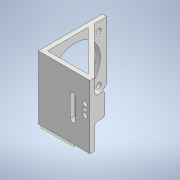
# Autodesk Inventor part: Bending Base
Saved by Autodesk Inventor 2022.2 (Build 262287000, 287)
## iProperties
Created: 2022-08-12
Part Number: Bending Base
Material: Generic
Document SubType Name: Modeling
Designer: Ilewicz
Density: 1 g/cm^3
Appearance: Default
Author: Ilewicz
Autodesk Inventor part; units mm, degrees
sketch "Sketch2" plane through (0, 0, 0) normal (1, 0, 0) x (0, 1, 0)
  line L0 (21.15, -4.6284) -> (21.15, -37.6716) projected
  line L1 (17.5822, -41.3607) -> (20.2107, -38.7322) projected
  arc A0 (20.2107, -38.7322) -> (20.65, -37.6716) centre (19.15, -37.6716) ccw projected
  line L2 (20.65, -37.6716) -> (20.65, -4.6284) projected
  arc A1 (20.65, -4.6284) -> (20.2107, -3.5678) centre (19.15, -4.6284) ccw projected
  line L3 (20.2107, -3.5678) -> (17.5822, -0.9393) projected
  arc A2 (17.5822, -0.9393) -> (16.5216, -0.5) centre (16.5216, -2) ccw projected
  line L4 (16.5216, -0.5) -> (-16.5216, -0.5) projected
  arc A3 (-16.5216, -0.5) -> (-17.5822, -0.9393) centre (-16.5216, -2) ccw projected
  line L5 (-17.5822, -0.9393) -> (-20.2107, -3.5678) projected
  arc A4 (-20.2107, -3.5678) -> (-20.65, -4.6284) centre (-19.15, -4.6284) ccw projected
  line L6 (-20.65, -4.6284) -> (-20.65, -37.6716) projected
  arc A5 (-20.65, -37.6716) -> (-20.2107, -38.7322) centre (-19.15, -37.6716) ccw projected
  line L7 (-20.2107, -38.7322) -> (-17.5822, -41.3607) projected
  arc A6 (-17.5822, -41.3607) -> (-16.5216, -41.8) centre (-16.5216, -40.3) ccw projected
  line L8 (-16.5216, -41.8) -> (16.5216, -41.8) projected
  arc A7 (16.5216, -41.8) -> (17.5822, -41.3607) centre (16.5216, -40.3) ccw projected
  circle A8 centre (0, -21.15) radius 16.5 projected
  circle A9 centre (15.5, -36.65) radius 1.55 projected
  circle A10 centre (-15.5, -36.65) radius 1.55 projected
  circle A11 centre (-15.5, -5.65) radius 1.55 projected
  circle A12 centre (15.5, -5.65) radius 1.55 projected
  line L9 (21.15, -37.6716) -> (21.15, -41.8)
  line L10 (21.15, -41.8) -> (15.1388, -41.8)
  line L11 (21.15, -4.6284) -> (21.15, -0.5)
  line L12 (-20.65, -4.7869) -> (-20.65, 0.2131)
  line L13 (-20.65, 0.2131) -> (21.15, 0.2131)
  line L14 (21.15, 0.2131) -> (21.15, -0.5)
  line L15 (-20.65, -4.7869) -> (-20.65, -4.6284)
  line L16 (21.15, -0.5) -> (20.65, -0.5)
  point P0 (0, 0)
  dimension "d2" = 5
  constraints: 16 end point, 3 vertical, 2 collinear, 2 point on line, 1 parallel
  measures "d2" distance of L12.start L12.end
extrude "Extrusion1" add sketch "Sketch2" along normal blind 3
sketch "Sketch5" plane through (3, 0, 0) normal (1, 0, 0) x (0, 0, -1)
  line L0 (41.8, 21.15) -> (-0.2131, 21.15) projected
  line L1 (-0.2131, -20.65) -> (37.6716, -20.65) projected
  line L2 (-0.2131, 21.15) -> (2.7869, 21.15)
  line L3 (2.7869, 21.15) -> (2.7869, -20.65)
  line L4 (2.7869, -20.65) -> (-0.2131, -20.65)
  line L5 (-0.2131, -20.65) -> (-0.2131, 21.15)
  point P0 (0, 0)
  dimension "d3" = 3
  constraints: 8 end point, 2 parallel, 1 horizontal, 1 perpendicular, 1 point on line
  measures "d3" distance of L3.end L4.end
ref_plane "Work Plane1" through (33.9341, -3.4404, -22.9827) normal (1, 0, 0) x (0, 1, 0)
extrude "Extrusion2" add sketch "Sketch5" along normal up to surface (30.9341 mm away)
sketch "Sketch12" plane through (0, 21.15, 0.2131) normal (0, 1, 0) x (1, 0, 0)
  line L0 (3, 3) -> (33.9341, 3) projected
  line L1 (29.6915, 3) -> (3, 29.6915)
  line L2 (3, 42.0131) -> (3, 3) projected
  line L3 (33.9341, 3) -> (3, 33.9341)
  line L4 (0, 42.0131) -> (0, 0) projected
  line L5 (0, 0) -> (33.9341, 0) projected
  line L6 (33.9341, 0) -> (33.9341, 3) projected
  line L7 (3, 3) -> (33.9341, 3) projected
  line L8 (3, 42.0131) -> (3, 3) projected
  line L9 (0, 42.0131) -> (3, 42.0131) projected
  point P0 (0, 0.2131)
  dimension "d25" = 3
  dimension "d26" = 45
  constraints: 4 end point, 3 point on line, 1 parallel
  measures "d25" distance between parallel lines of L1 L3
  measures "d26" angle of L2 L1
extrude "Extrusion7" add sketch "Sketch12" against normal blind 2 contours L0 L6 L5 L4 L9 L2 | L1 L2 L3 L0
ref_plane "Work Plane6" through (28.6495, -6.0754, -9.5607) normal (0, 0, 1) x (1, 0, 0)
sketch "Sketch7" plane through (3, -20.65, -2.7869) normal (0, 0, -1) x (-1, 0, 0)
  line L0 (-28.65, 23.05) -> (-28.65, 21.7895) projected
  arc A0 (-28.65, 23.05) -> (-28.25, 22.65) centre (-28.25, 23.05) ccw projected
  line L1 (-28.25, 22.65) -> (-25.65, 22.65) projected
  line L2 (-25.65, 15.5156) -> (-25.65, 22.65) projected
  line L3 (-25.65, 15.5156) -> (-27.64, 17.5537) projected
  line L4 (-27.64, 17.5537) -> (-27.65, 17.5537) projected
  line L5 (-29.9084, 20.2451) -> (-27.65, 17.5537) projected
  ellipse E0 centre (-29.15, 20.9127) end of major axis (-29.15, 19.8885) minor radius 1 (-30.15, 20.9127) -> (-29.9084, 20.2451) ccw projected
  line L6 (-30.15, 21.0006) -> (-30.15, 20.9127) projected
  line L7 (-30.15, 27.15) -> (-30.15, 21.0006) projected
  line L8 (-30.15, 27.15) -> (-28.65, 27.15) projected
  line L9 (-28.65, 21.7895) -> (-28.65, 27.15) projected
  line L10 (0, 0) -> (-30.9341, 0) projected
  line L11 (-25.65, 0) -> (-25.65, 41.8)
  line L12 (0, 41.8) -> (-30.9341, 41.8) projected
  line L13 (-30.9341, 39.8) -> (-30.9341, 0) projected
  line L14 (0, 0) -> (-30.9341, 0) projected
  line L15 (0, 41.8) -> (0, 0) projected
  line L16 (0, 41.8) -> (-26.6915, 41.8) projected
  circle A1 centre (-27.6209, 23.6216) radius 1.25
  circle A2 centre (-27.653, 20.3029) radius 1.5 projected
  circle A3 centre (-27.653, 26.8687) radius 1.5 projected
  line L17 (-26.6915, 41.8) -> (-26.6915, 39.8) projected
  line L18 (-26.6915, 39.8) -> (-30.9341, 39.8) projected
  line L19 (-30.9341, 2) -> (-30.9341, 0) projected
  line L20 (-30.9341, 41.8) -> (-30.9341, 39.8) projected
  line L21 (-25.65, 31.1874) -> (-30.9341, 31.1874)
  line L22 (-30.9341, 39.8) -> (-30.9341, 0) projected
  line L23 (-25.65, 16.0384) -> (-30.9341, 16.0384)
  point P0 (3, 20.65)
  point P1 (-30.9341, 19.4722)
  point P2 (-30.9341, 0)
  point P3 (-30.9341, 41.8)
  point P4 (-30.9341, 23.8955)
  point P5 (-30.9341, 19.4722)
  point P6 (-25.65, 15.5156)
  point P7 (-25.65, 22.65)
  point P8 (-25.65, 41.8)
  point P9 (-30.9341, 25.7096)
  point P10 (-30.9341, 17.4244)
  point P11 (-30.9341, 16.0384)
  point P12 (-25.65, 16.0384)
  point P13 (-26.1605, 16.0384)
  point P14 (-29.1264, 27.15)
  point P15 (-28.65, 25.748)
  point P16 (-28.65, 24.3312)
  point P17 (-26.8345, 22.65)
  dimension "d23" = 2.5
  constraints: 6 end point, 6 point on line, 2 perpendicular, 1 centre point, 1 collinear, 1 tangent, 1 vertical, 1 other
  measures "d23" diameter of A1
extrude "Extrusion3" add sketch "Sketch7" along normal up to surface (6.7738 mm away) contours A1 L1 L2 L23 L3 L4 L5 E0 L6 L7 L8 A3 L9 | L9 A3 L8 L7 L6 E0 L5 L4 L3 L23 L13 L21 L11 L1 A1
ref_plane "Work Plane5" through (3, -20.65, -9.2979) normal (0, 0, -1) x (-1, 0, 0)
sketch "Sketch10" plane through (0, -20.65, 0.2131) normal (0, 0, 1) x (1, 0, 0)
  circle A0 centre (22.5901, 16.9163) radius 1.59 projected
  circle A1 centre (22.5901, 25.2418) radius 1.59 projected
  line L0 (24.1801, 28.0246) -> (24.1801, 13.7754)
  line L1 (21.0001, 13.7754) -> (21.0001, 28.0246)
  arc A2 (21.0001, 13.7754) -> (24.1801, 13.7754) centre (22.5901, 13.7754) ccw
  line L2 (3, 0) -> (32.7496, 13.2856) projected
  arc A3 (24.1801, 28.0246) -> (21.0001, 28.0246) centre (22.5901, 28.0246) ccw
  line L3 (33.9341, 27.9855) -> (3, 41.8) projected
  point P0 (0, 20.65)
  point P1 (32.8942, 25.4407)
  point P2 (3, 41.8)
  point P3 (33.9341, 27.9855)
  dimension "d16" = 4.59
  dimension "d17" = 4.59
  constraints: 5 tangent, 4 end point, 4 point on circle, 2 centre point, 2 equal radius, 1 vertical, 1 other
  measures "d16" distance from line of L2 A2.centre
extrude "Extrusion5" cut sketch "Sketch10" against normal blind 10
ref_plane "Work Plane3" through (20.0901, -24.2569, 0.2131) normal (0, -1, 0) x (1, 0, 0)
sketch "Sketch14" plane through (33.9341, -20.65, 0.2131) normal (1, 0, 0) x (0, 0, -1)
  point P0 (0.2131, 20.65)
sketch "Sketch15" plane through (33.9341, -20.65, -9.5607) normal (0, 0, -1) x (-1, 0, 0)
  circle A0 centre (3.2811, 20.3029) radius 1.5 projected
  circle A1 centre (3.2811, 20.3029) radius 1.5 projected
  circle A2 centre (3.3132, 23.6216) radius 1.25 projected
  circle A3 centre (3.2811, 26.8687) radius 1.5 projected
  circle A4 centre (3.2811, 20.3029) radius 1.5 projected
  line L0 (0, 16.0384) -> (5.2841, 16.0384) projected
  line L1 (5.2841, 16.0384) -> (5.2841, 31.1874) projected
  line L2 (5.2841, 31.1874) -> (0, 31.1874) projected
  line L3 (0, 31.1874) -> (0, 16.0384) projected
  point P0 (33.9341, 20.65)
extrude "Extrusion9" cut sketch "Sketch15" against normal through all contours A0 | A2 | A3
sketch "Sketch16" plane through (0, -20.65, -37.6716) normal (0, -1, 0) x (1, 0, 0)
  line L0 (0, 37.8846) -> (0, 0) projected
  line L1 (0, 0) -> (3, 0) projected
  line L2 (3, 34.8846) -> (3, 0) projected
  line L3 (3, 34.8846) -> (33.9341, 34.8846) projected
  line L4 (0, 37.8846) -> (33.9341, 37.8846) projected
  line L5 (29.6915, 34.8846) -> (3, 8.1932) projected
  line L6 (3, 3.9505) -> (3, 8.1932) projected
  line L7 (3, 3.9505) -> (33.9341, 34.8846) projected
  line L8 (29.6915, 34.8846) -> (33.9341, 34.8846) projected
  line L9 (33.9341, 34.8846) -> (33.9341, 37.8846) projected
  point P0 (0, 37.6716)
  point P1 (3, 8.1932)
extrude "Extrusion10" add sketch "Sketch16" against normal blind 2 contours L7 L2 L5 L3
fillet "Fillet3" radius 2 4 edges at (31.292, 10.5374, -9.5607) (31.292, 10.5374, -2.7869) (31.292, -4.6116, -9.5607) (31.292, -4.6116, -2.7869)
body "Solid1"
